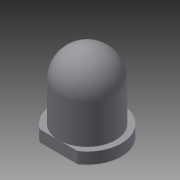
# Autodesk Inventor part: led
Saved by Autodesk Inventor 2015 (Build 190159000, 159)
## iProperties
Created: 2014-08-01
Part Number: led
Material: Generic
Document SubType Name: Modeling
Designer: dan
Density: 1 g/cm^3
Appearance: Default
Author: dan
Autodesk Inventor part; units mm, degrees
ref_plane "YZ Plane" through (0, 0, 0) normal (1, 0, 0) x (0, 1, 0)
ref_plane "XZ Plane" through (0, 0, 0) normal (0, 1, 0) x (-1, 0, 0)
ref_plane "XY Plane" through (0, 0, 0) normal (0, 0, 1) x (1, 0, 0)
sketch "Sketch1" plane through (0, 0, 0) normal (0, 0, 1) x (1, 0, 0)
  line L0 (22.225, 0) -> (30.48, 0)
  line L1 (30.48, 0) -> (30.48, 10.16)
  line L2 (30.48, 10.16) -> (25.4, 10.16)
  line L3 (25.4, 10.16) -> (25.4, 44.45)
  line L4 (25.4, 44.45) -> (0, 44.45) construction
  line L5 (0, 10.16) -> (0, 0)
  arc A0 (25.4, 44.45) -> (0, 69.85) centre (0, 44.45) ccw
  line L6 (0, 66.675) -> (0, 69.85)
  arc A1 (22.225, 44.45) -> (0, 66.675) centre (0, 44.45) ccw
  line L7 (22.225, 44.45) -> (22.225, 0)
  line L8 (0, 66.675) -> (0, 0) construction
  line L9 (0, 0) -> (22.225, 0) construction
  dimension "d2" = 3.175
  dimension "d3" = 10.16
  dimension "d4" = 69.85
  dimension "d6" = 25.4
  dimension "d7" = 5.08
  constraints: 20 end point, 6 perpendicular, 4 point on circle, 2 centre point, 2 horizontal, 2 line through centre, 2 vertical, 1 coincident, 1 point on line, 1 tangent
  measures "d2" distance between parallel lines of L3 L7
  measures "d3" distance of L0.end L1.end
  measures "d4" distance of L5.end L6.end
  measures "d6" distance between parallel lines of L8 L3
  measures "d7" distance of L1.end L2.end
revolve "Revolution1" add sketch "Sketch1" angle 360 about axis through (0, 66.675, 0) along (0, -1, 0)
sketch "Sketch3" plane through (0, 0, 0) normal (0, -1, 0) x (1, 0, 0)
  circle A0 centre (0, 0) radius 25.4 construction
  circle A1 centre (0, 0) radius 30.48 projected
  line L0 (0, 25.4) -> (-16.8485, 25.4)
  line L1 (0, 25.4) -> (16.8485, 25.4)
  arc A2 (-16.8485, 25.4) -> (0, 30.48) centre (0, 0) ccw
  constraints: 6 point on circle, 4 end point, 1 centre point, 1 concentric, 1 horizontal, 1 point on line, 1 vertical alignment, 1 other
extrude "Extrusion1" cut sketch "Sketch3" against normal up to next contours L1 L0 A1 picked at (-9.4832, 26.3286)
sketch "Sketch4" plane through (0, 0, 0) normal (0, -1, 0) x (1, 0, 0)
  arc A0 (-18.7397, -4.725) -> (-18.7397, 4.725) centre (-18.7397, 0) ccw
  circle A1 centre (-18.7397, 0) radius 1.55
  line L0 (-18.7397, 4.725) -> (-21.7169, 4.725)
  line L1 (-18.7397, -4.725) -> (-21.7169, -4.725)
  arc A2 (-21.7169, 4.725) -> (-21.7169, -4.725) centre (0, 0) ccw
  point P0 (0, 0)
  dimension "d13" = 3.1
  dimension "d14" = 3.175
  constraints: 4 end point, 4 point on circle, 3 centre point, 2 horizontal, 2 tangent, 1 coincident
  measures "d13" diameter of A1
  measures "d14" radial gap between concentric circles of A0 A1
extrude "Extrusion2" add sketch "Sketch4" against normal blind 9.652
pattern_circular "Circular Pattern1" count 4 over 360 about axis through (0, 27.305, 0) along (0, -1, 0) of "Extrusion2"
body "Solid1"
